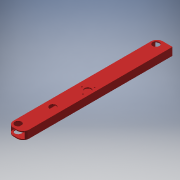
# Autodesk Inventor part: arm
Saved by Autodesk Inventor 2017 SP1 (Build 210196100, 196)
## iProperties
Created: 2018-01-23
Part Number: arm
Material: Aluminum 6061
Document SubType Name: Modeling
Designer: Ben
Density: 2.7 g/cm^3
Appearance: Light Red
Mass: 549.113 g
Surface Area: 1310.83 cm^2
Volume: 203.375 cm^3
Author: Ben
Autodesk Inventor part; units mm, degrees
ref_plane "YZ Plane" through (0, 0, 0) normal (1, 0, 0) x (0, 1, 0)
ref_plane "XZ Plane" through (0, 0, 0) normal (0, 1, 0) x (-1, 0, 0)
ref_plane "XY Plane" through (0, 0, 0) normal (0, 0, 1) x (1, 0, 0)
sketch "Sketch1" plane through (0, 0, 0) normal (0, 0, 1) x (1, 0, 0)
  line L0 (-25.4, -12.7) -> (25.4, -12.7)
  line L1 (25.4, -12.7) -> (25.4, 12.7)
  line L2 (25.4, 12.7) -> (-25.4, 12.7)
  line L3 (-25.4, 12.7) -> (-25.4, -12.7)
  line L4 (-25.4, -12.7) -> (25.4, 12.7) construction
  line L5 (25.4, -12.7) -> (-25.4, 12.7) construction
  line L6 (-22.225, -9.525) -> (22.225, -9.525)
  line L7 (22.225, -9.525) -> (22.225, 9.525)
  line L8 (22.225, 9.525) -> (-22.225, 9.525)
  line L9 (-22.225, 9.525) -> (-22.225, -9.525)
  line L10 (-22.225, -9.525) -> (22.225, 9.525) construction
  line L11 (22.225, -9.525) -> (-22.225, 9.525) construction
  line L12 (0, 9.525) -> (0, 12.7) construction
  line L13 (22.225, 0) -> (25.4, 0) construction
  point P0 (0, 0)
  dimension "d0" = 25.4
  dimension "d1" = 50.8
  dimension "d2" = 3.175
  constraints: 28 end point, 8 midpoint, 4 parallel, 3 perpendicular, 2 horizontal
  measures "d0" distance of L0.end L1.end
  measures "d1" distance of L1.end L2.end
  measures "d2" distance of L12.start L12.end
extrude "Extrusion1" add sketch "Sketch1" along normal blind 488.95
sketch "Sketch2" plane through (-25.4, 12.7, 0) normal (0, 1, 0) x (1, 0, 0)
  circle A0 centre (15.875, -469.9) radius 11.1125
  circle A1 centre (34.925, -261.2177) radius 11.1125
  circle A2 centre (25.4, -365.5589) radius 11.1125
  circle A3 centre (15.875, -19.05) radius 11.1125
  line L0 (0, 0) -> (0, -488.95) construction
  line L1 (3.175, 0) -> (3.175, -488.95) construction
  line L2 (50.8, 0) -> (50.8, -488.95) construction
  line L3 (15.875, -19.05) -> (24.1367, -26.4818) construction
  line L4 (15.875, -469.9) -> (34.925, -261.2177) construction
  line L5 (50.8, -488.95) -> (0, -488.95) projected
  line L6 (47.625, 0) -> (47.625, -488.95) construction
  circle A4 centre (41.275, -242.1677) radius 1.905
  circle A5 centre (41.275, -280.2677) radius 1.905
  circle A6 centre (12.7, -261.2177) radius 1.905
  line L7 (41.275, -242.1677) -> (41.275, -280.2677) construction
  line L8 (12.7, -261.2177) -> (47.625, -261.2177) construction
  circle A7 centre (34.925, -261.2177) radius 14.2875 construction
  point P0 (41.275, -261.2177)
  dimension "d10" = 22.225
  dimension "d5" = 22.225
  dimension "d7" = 209.55
  dimension "d16" = 19.05
  dimension "d17" = 15.875
  dimension "d20" = 19.05
  dimension "d21" = 15.875
  dimension "d23" = 15.875
  dimension "d24" = 38.1
  dimension "d27" = 28.575
  dimension "d28" = 3.81
  dimension "d29" = 22.225
  dimension "d30" = 9.525
  constraints: 8 end point, 7 centre point, 4 equal radius, 3 point on line, 2 coincident, 2 midpoint, 1 parallel, 1 perpendicular, 3 other
  measures "d5" diameter of A0
  measures "d7" distance of L4.start L4.end
  measures "d16" vertical distance of L3.start L0.start
  measures "d17" distance from line of L0 L4.start
  measures "d20" distance from line of L5 L4.start
  measures "d21" distance from line of L0 L3.start
  measures "d23" distance from line of L2 L4.end
  measures "d24" distance of L7.start L7.end
  measures "d27" diameter of A7
  measures "d28" diameter of A6
  measures "d29" distance of L4.end L8.start
  measures "d30" distance between parallel lines of L2 L7
extrude "Extrusion2" cut sketch "Sketch2" against normal through all
fillet "Fillet1" radius 19.05 3 edges at (-25.4, 0, 0) (-25.4, 0, 488.95) (25.4, 0, 488.95)
body "Solid1"
